Autodesk Inventor part; units mm, degrees
(part 2 of 2)
sketch "Sketch25" plane through (28.3887, -28.3887, -12.2281) normal (0.3845744, -0.3845744, 0.8391693) x (0.7071068, 0.7071068, 0)
  line L0 (-5, 5.9354) -> (-10.5804, 16.196) projected
  line L1 (-5, 0) -> (-5, 5.9354) projected
  line L2 (0, 0) -> (-5, 0) projected
  line L3 (0, 16.196) -> (0, 0) projected
  line L4 (0, 16.196) -> (-10.5804, 16.196) projected
  line L5 (0, 0) -> (5, 0)
  line L6 (0, 0) -> (5, 0) construction
  line L7 (0, 16.196) -> (0, 13.696)
  line L8 (0, 0) -> (0, 1)
  line L9 (0, 1) -> (5, 1)
  line L10 (5, 1) -> (0, 13.696)
  point P0 (0, 40.3412)
  dimension "d119" = 5
  dimension "d120" = 0
  dimension "d121" = 16.196
  dimension "d122" = 2.5
  dimension "d123" = 1
  constraints: 12 end point, 2 horizontal, 2 point on line, 1 collinear, 1 perpendicular
  measures "d119" distance of L2.start L5.end
  measures "d120" distance between parallel lines of L5 L6
  measures "d121" distance of L3.start L2.start
  measures "d122" distance of L3.start L7.end
  measures "d123" distance of L2.start L8.end
extrude "Extrusion25" [suppressed]
sketch "Sketch26" plane through (36.3604, -56.1594, -27.5) normal (0, 0, -1) x (-1, 0, 0)
  line L0 (-6.364, 6.364) -> (38.7544, 51.4823) projected
  line L1 (22.18, 34.9079) -> (23.9685, 35.2898) projected
  line L2 (25.2724, 28.9217) -> (13.7291, 26.457) projected
  line L3 (23.9685, 35.2898) -> (25.3827, 36.704)
  line L4 (13.7291, 26.457) -> (12.3149, 25.0428)
  line L5 (25.2724, 28.9217) -> (26.6866, 27.5075)
  line L6 (24.6794, 37.4073) -> (12.3149, 25.0428)
  line L7 (12.3149, 25.0428) -> (18.2684, 19.0892)
  line L8 (18.2684, 19.0892) -> (30.6329, 31.4538)
  line L9 (30.6329, 31.4538) -> (24.6794, 37.4073)
  line L10 (198.4388, -108.2021) -> (153.3204, -153.3204) projected
  line L11 (24.6794, 37.4073) -> (12.3149, 25.0428)
  line L12 (12.3149, 25.0428) -> (171.9993, -134.6416)
  line L13 (171.9993, -134.6416) -> (184.3638, -122.2771)
  line L14 (184.3638, -122.2771) -> (24.6794, 37.4073)
  point P0 (36.3604, 56.1594)
  point P1 (184.3638, -122.2771)
  point P2 (30.6329, 31.4538)
  point P3 (18.2684, 19.0892)
  dimension "d126" = 2
  dimension "d127" = 2
  dimension "d128" = 2
  constraints: 22 end point, 4 parallel, 2 perpendicular, 2 point on line, 1 collinear
  measures "d126" distance of L1.end L3.end
  measures "d127" distance of L2.end L4.end
  measures "d128" distance of L2.start L5.end
ref_plane "Work Plane11" through (-136.5618, -189.878, -16.0044) normal (-0.3845744, 0.3845744, -0.8391693) x (-0.7071068, -0.7071068, 0)
sketch "Sketch27" plane through (-136.5618, -189.878, -16.0044) normal (-0.3845744, 0.3845744, -0.8391693) x (-0.7071068, -0.7071068, 0)
  line L0 (5, 16.2505) -> (5, 0) projected
  line L1 (5, 16.2505) -> (5, 13.7505)
  line L2 (5, 0) -> (5, 1)
  line L3 (5, 1) -> (10, 1)
  line L4 (10, 1) -> (5, 13.7505)
  point P0 (-230.8278, 40.3412)
  dimension "d131" = 2.5
  dimension "d132" = 1
  dimension "d133" = 5
  dimension "d134" = 90
  constraints: 8 end point, 2 point on line, 1 perpendicular
  measures "d131" distance of L0.start L1.end
  measures "d132" distance of L0.end L2.end
  measures "d133" distance of L2.end L3.end
  measures "d134" angle of L2 L3
ref_plane "Work Plane6" through (23.1226, -30.1936, -16.0044) normal (-0.3845744, 0.3845744, -0.8391693) x (-0.7071068, -0.7071068, 0)
sketch "Sketch28" plane through (23.1226, -30.1936, -16.0044) normal (-0.3845744, 0.3845744, -0.8391693) x (-0.7071068, -0.7071068, 0)
  line L0 (-5, 13.696) -> (-5, 16.2505) projected
  line L1 (-5, 13.696) -> (-10, 1) projected
  line L2 (-5, 16.2505) -> (-4.129, 15.9075)
  line L3 (-5, 16.2505) -> (0, 16.2505) projected
  line L4 (-6.3009, 10.3927) -> (-3.994, 16.2505)
  point P0 (-5, 40.3412)
  point P1 (-5, 13.696)
  constraints: 4 end point, 2 point on line
ref_plane "Work Plane4" through (18.0345, -19.4573, -3.3899) normal (-0.3845744, 0.3845744, -0.8391693) x (-0.5933823, 0.5933823, 0.5438703)
sketch "Sketch29" plane through (18.0345, -19.4573, -3.3899) normal (-0.3845744, 0.3845744, -0.8391693) x (-0.5933823, 0.5933823, 0.5438703)
  line L0 (-0.0545, 1.006) -> (-0.0545, 0.0215) projected
  line L1 (0, 0) -> (-0.0545, 0.0215) projected
  line L2 (0, 1.006) -> (0, 0) projected
  line L3 (-0.0545, 1.006) -> (0, 1.006) projected
  line L4 (-0.0545, -3.994) -> (-17.2505, -3.994) construction
  line L5 (-16.2505, -3.994) -> (-0.0545, -3.994) construction
  line L6 (-0.0545, 1.006) -> (0, 1.006)
  line L7 (0, 1.006) -> (0, -3.994)
  line L8 (0, -3.994) -> (-0.0545, -3.994)
  line L9 (-0.0545, -3.994) -> (-0.0545, 1.006)
  point P0 (24.0907, 1.006)
  constraints: 8 end point, 2 parallel, 1 horizontal, 1 perpendicular
sketch "Sketch31" plane through (-0.9798, 0.9798, -25.5) normal (0.7071068, 0.7071068, 0) x (-0.7071068, 0.7071068, 0)
  line L0 (-27.9421, 22.0804) -> (-28.486, 22.9196) projected
  line L1 (-25.4489, 18.3338) -> (-24.9051, 17.4947) projected
  line L2 (-42.9163, 13.5672) -> (-28.486, 22.9196) projected
  line L3 (-28.486, 22.9196) -> (-28.4402, 22.9493)
  line L4 (-28.4402, 22.9493) -> (-27.8964, 22.1101)
  line L5 (-27.8964, 22.1101) -> (-27.9421, 22.0804)
  line L6 (-27.9421, 22.0804) -> (-28.486, 22.9196)
  point P0 (-1.3856, 25.5)
  point P1 (-27.8964, 22.1101)
  constraints: 8 end point, 2 parallel, 2 perpendicular
ref_plane "Work Plane10" through (23.1226, -30.1936, -16.0044) normal (-0.3845744, 0.3845744, -0.8391693) x (-0.7071068, -0.7071068, 0)
sketch "Sketch32" plane through (23.1226, -30.1936, -16.0044) normal (-0.3845744, 0.3845744, -0.8391693) x (-0.7071068, -0.7071068, 0)
  line L0 (-5, 13.696) -> (-10, 1) projected
  line L1 (-10, 1) -> (-5, 1) projected
  line L2 (-5, 0) -> (-5, 1) projected
  line L3 (-5, 0) -> (0, 0) projected
  line L4 (0, 12.8787) -> (0, 0) projected
  line L5 (-5, 16.2505) -> (1.8338, 16.2505) projected
  line L6 (-5, 13.696) -> (-10, 1) projected
  line L7 (0, 16.2505) -> (0, 0) projected
  line L8 (0, 16.2505) -> (0, 11.2505)
  line L9 (-3.994, 16.2505) -> (-2.494, 16.2505)
  line L10 (-5, 16.2505) -> (0, 16.2505) projected
  line L11 (0, 11.2505) -> (-2.494, 16.2505)
  line L12 (-2.494, 16.2505) -> (-2.494, 11.2505)
  line L13 (-2.494, 16.2505) -> (2.506, 16.2505) construction
  line L14 (-2.494, 11.2505) -> (0, 11.2505)
  line L15 (225.8278, 0) -> (225.8278, 12.8787) projected
  line L16 (225.8278, 0) -> (230.8278, 0) projected
  line L17 (230.8278, 16.2505) -> (230.8278, 0) projected
  line L18 (223.994, 16.2505) -> (230.8278, 16.2505) projected
  line L19 (-5, 13.696) -> (-5, 16.2505) projected
  line L20 (225.8278, 12.8787) -> (223.994, 16.2505) projected
  line L21 (1.8338, 16.2505) -> (0, 12.8787) projected
  point P0 (-5, 40.3412)
  point P1 (-2.494, 16.2505)
  point P2 (0, 11.2505)
  dimension "d144" = 5
  dimension "d145" = 1.5
  dimension "d148" = 5
  dimension "d149" = 90
  constraints: 12 end point, 2 perpendicular, 2 point on line, 1 horizontal
  measures "d144" distance of L7.start L8.end
  measures "d145" distance of L9.start L9.end
  measures "d148" distance of L9.end L12.end
  measures "d149" angle of L12 L13
ref_plane "Work Plane3" through (15.2433, -18.7874, -7.1662) normal (-0.7071068, -0.7071068, 0) x (-0.3845744, 0.3845744, -0.8391693)
sketch "Sketch33" plane through (15.2433, -18.7874, -7.1662) normal (-0.7071068, -0.7071068, 0) x (-0.3845744, 0.3845744, -0.8391693)
  line L0 (-4.5, 0) -> (-4.5, 5) projected
  line L1 (-4.5, 5) -> (0, 5) projected
  line L2 (0, 5) -> (0, 0) projected
  line L3 (-5.5, 0) -> (1, 0) projected
  line L4 (-12.0423, 10.0013) -> (-2.5322, -4.6725) projected
  line L5 (-5.5, 0) -> (-5.5, 17.2505) projected
  line L6 (-5.5, 0) -> (-5.5, -0.0933)
  line L7 (-5.5, 0) -> (-5.4067, 0) construction
  line L8 (1, 0) -> (1, 17.2505) projected
  line L9 (2.9224, -1.1374) -> (-2.5322, -4.6725) projected
  line L10 (1, 0) -> (1, -2.6217)
  line L11 (1, 0) -> (3.6217, 0) construction
  line L12 (2.5, 17.2505) -> (2.5, -1.5)
  line L13 (2.5, -1.5) -> (-7, -1.5)
  line L14 (-7, -1.5) -> (-7, 17.2505)
  point P0 (7.0737, -24.0907)
  point P1 (-4.5883, -1.5)
  point P2 (1, -1.5)
  dimension "d150" = 90
  dimension "d151" = 90
  dimension "d152" = 1.5
  constraints: 14 end point, 2 horizontal, 2 perpendicular, 1 point on line, 2 other
  measures "d150" angle of L6 L7
  measures "d151" angle of L10 L11
  measures "d152" distance between parallel lines of L3 L13
ref_plane "Work Plane8" through (-136.5618, -189.878, -16.0044) normal (-0.3845744, 0.3845744, -0.8391693) x (-0.7071068, -0.7071068, 0)
sketch "Sketch35" plane through (-136.5618, -189.878, -16.0044) normal (-0.3845744, 0.3845744, -0.8391693) x (-0.7071068, -0.7071068, 0)
  line L0 (0, 16.2505) -> (5, 16.2505) projected
  line L1 (5, 16.2505) -> (5, 0) projected
  line L2 (10, 1) -> (5, 13.7505) projected
  line L3 (7.0437, 8.539) -> (4.0196, 16.2505)
  point P0 (-230.8278, 40.3412)
  point P1 (5, 13.7505)
  constraints: 2 end point, 2 point on line
sketch "Sketch36" plane through (-205.4791, -128.0318, -8.9699) normal (-0.7071068, -0.7071068, 0) x (-0.7071068, 0.7071068, 0)
  line L0 (-81.8639, -6.3895) -> (-96.2942, 2.9629) projected
  line L1 (-78.283, -0.9645) -> (-78.8268, -1.8037) projected
  line L2 (-81.8639, -6.3895) -> (-81.32, -5.5503)
  line L3 (-81.32, -5.5503) -> (-81.2742, -5.58)
  line L4 (-81.2742, -5.58) -> (-81.8181, -6.4191)
  line L5 (-81.8181, -6.4191) -> (-81.8639, -6.3895)
  point P0 (-54.7635, -8.9699)
  point P1 (-81.2742, -5.58)
  constraints: 8 end point, 2 parallel, 1 perpendicular
sketch "Sketch37" plane through (-116.96, -209.4798, -27.5) normal (0.7071068, 0.7071068, 0) x (-0.7071068, 0.7071068, 0)
  line L0 (38.9106, 24.1101) -> (34.7148, 21.3907) projected
  line L1 (41.3581, 20.3338) -> (38.9106, 24.1101) projected
  line L2 (37.1622, 17.6145) -> (41.3581, 20.3338) projected
  line L3 (37.1622, 17.6145) -> (34.7148, 21.3907) projected
  point P0 (65.4214, 27.5)
sketch "Sketch38" plane through (-113.5512, 93.7522, -27.5) normal (0, 0, -1) x (-1, 0, 0)
  line L0 (-69.1707, -56.4428) -> (-6.364, 6.364) projected
  line L1 (-21.6597, -8.9317) -> (-23.6391, -19.8047) projected
  line L2 (-30.0242, -18.5868) -> (-29.737, -17.0091) projected
  line L3 (-29.0404, -18.7659) -> (-30.0242, -18.5868) projected
  line L4 (-30.0242, -18.5868) -> (-30.6695, -17.9415)
  line L5 (-30.6695, -17.9415) -> (-31.3766, -18.6487)
  line L6 (-21.6597, -8.9317) -> (-20.9525, -8.2246)
  line L7 (-20.9525, -8.2246) -> (-31.3766, -18.6487)
  line L8 (-31.3766, -18.6487) -> (128.3078, -178.3331)
  line L9 (128.3078, -178.3331) -> (138.7319, -167.909)
  line L10 (138.7319, -167.909) -> (-20.9525, -8.2246)
  point P0 (-113.5512, -93.7522)
  dimension "d174" = 1
  dimension "d175" = 1
  constraints: 14 end point, 3 point on line, 2 parallel, 2 perpendicular, 1 collinear
  measures "d174" distance of L4.end L5.end
  measures "d175" distance of L1.start L6.end
ref_plane "Work Plane7" through (-244.7474, -81.6925, -3.5337) normal (-0.4023607, 0.4023607, 0.8223209) x (0.7071068, 0.7071068, 0)
sketch "Sketch39" plane through (-244.7474, -81.6925, -3.5337) normal (-0.4023607, 0.4023607, 0.8223209) x (0.7071068, 0.7071068, 0)
  line L0 (-5, 0) -> (-5, 16.2505) projected
  line L1 (-5, 16.2505) -> (-5, 15.2505)
  line L2 (-5, 15.2505) -> (-10, 15.2505)
  line L3 (-10, 15.2505) -> (-5, 0)
  line L4 (-5, 15.2505) -> (-5, 14.2505)
  line L5 (-5, 14.2505) -> (-9.6721, 14.2505)
  point P0 (230.8278, -96.8221)
  dimension "d178" = 1
  dimension "d179" = 5
  dimension "d180" = 90
  dimension "d183" = 1
  constraints: 10 end point, 3 point on line, 2 perpendicular
  measures "d178" distance of L0.end L1.end
  measures "d179" distance of L1.end L2.end
  measures "d180" angle of L1 L2
  measures "d183" distance of L1.end L4.end
ref_plane "Work Plane5" through (-81.5274, 81.5274, -3.5337) normal (-0.4023607, 0.4023607, 0.8223209) x (0.7071068, 0.7071068, 0)
sketch "Sketch40" plane through (-81.5274, 81.5274, -3.5337) normal (-0.4023607, 0.4023607, 0.8223209) x (0.7071068, 0.7071068, 0)
  line L0 (0, 16.2505) -> (0, 0) projected
  line L1 (0, 16.2505) -> (-5, 16.2505) projected
  line L2 (0, 16.2505) -> (0, 15.2505)
  line L3 (0, 0) -> (0, 17.2505) projected
  line L4 (0, 15.2505) -> (5, 15.2505)
  line L5 (0, 0) -> (-10.4663, 0) projected
  line L6 (5, 15.2505) -> (0, 0)
  line L7 (0, 15.2505) -> (0, 14.2505)
  line L8 (0, 14.2505) -> (4.6721, 14.2505)
  point P0 (0, -96.8221)
  point P1 (-5, 0)
  point P2 (0, 14.2505)
  dimension "d184" = 1
  dimension "d185" = 5
  dimension "d186" = 90
  dimension "d187" = 1
  constraints: 10 end point, 3 point on line, 2 perpendicular
  measures "d184" distance of L0.start L2.end
  measures "d185" distance of L2.end L4.end
  measures "d186" angle of L4 L2
  measures "d187" distance of L2.end L7.end
sketch "Sketch41" plane through (-107.1872, 100.1162, -9) normal (-0.7071068, -0.7071068, 0) x (-0.7071068, 0.7071068, 0)
  line L0 (-33.8042, -1.7349) -> (-20.4859, 7.481) projected
  line L1 (-31.2884, -5.4663) -> (-17.9253, 3.7806) projected
  line L2 (-34.3732, -0.9125) -> (-33.8042, -1.7349) projected
  line L3 (-35.6067, -1.7661) -> (-34.1841, -3.8219)
  line L4 (-34.1841, -3.8219) -> (-19.6323, 6.2476)
  line L5 (-34.3732, -0.9125) -> (-35.6067, -1.7661)
  line L6 (-35.1718, -2.3945) -> (-32.3309, -6.5)
  line L7 (-20.6314, -6.5) -> (-35.3732, -6.5) projected
  line L8 (-16.5339, 3.5273) -> (-30.7194, -6.2887) projected
  line L9 (-30.07, -5.8393) -> (-31.0248, -6.5)
  line L10 (-35.6067, -1.7661) -> (-31.4951, 1.0791)
  line L11 (-31.4951, 1.0791) -> (-27.7964, -4.266)
  point P0 (-146.5856, -9)
  point P1 (-34.5078, -3.3541)
  dimension "d190" = 1.5
  dimension "d191" = 5
  constraints: 14 end point, 6 point on line, 2 perpendicular, 1 other
  measures "d190" distance between parallel lines of L2 L3
  measures "d191" distance of L3.start L10.end
sketch "Sketch43" plane through (-205.4791, -128.0318, -8.9699) normal (-0.7071068, -0.7071068, 0) x (-0.7071068, 0.7071068, 0)
  line L0 (-95.6027, 3.1105) -> (-16.2332, 125.5744)
  line L1 (-120.1849, 18.5301) -> (-55.3779, 18.5301) projected
  line L2 (-120.1849, -13.9699) -> (-120.1849, 18.5301) projected
  line L3 (91.8221, -13.9699) -> (-120.1849, -13.9699) projected
  line L4 (91.8221, 18.5301) -> (91.8221, -13.9699) projected
  line L5 (2, 18.5301) -> (91.8221, 18.5301) projected
  line L6 (0, 16.5301) -> (2, 18.5301) projected
  line L7 (0, 16.5301) -> (0, 0) projected
  line L8 (0, 0) -> (-5.4, 0) projected
  line L9 (-5.4, 0) -> (-5.4, 16.5301) projected
  line L10 (-7.4, 18.5301) -> (-5.4, 16.5301) projected
  line L11 (-45.9779, 18.5301) -> (-7.4, 18.5301) projected
  line L12 (-47.9779, 16.5301) -> (-45.9779, 18.5301) projected
  line L13 (-47.9779, 16.5301) -> (-47.9779, 0) projected
  line L14 (-47.9779, 0) -> (-53.3779, 0) projected
  line L15 (-53.3779, 0) -> (-53.3779, 16.5301) projected
  line L16 (-55.3779, 18.5301) -> (-53.3779, 16.5301) projected
  line L17 (-100.0531, 9.3651) -> (-100.0531, 4.1651) projected
  line L18 (-100.0531, 4.1651) -> (-110.4531, 4.1651) projected
  line L19 (-110.4531, 4.1651) -> (-110.4531, 9.3651) projected
  arc A0 (-100.0531, 9.3651) -> (-110.4531, 9.3651) centre (-105.2531, 9.3651) ccw projected
  line L20 (77.6221, 4.1651) -> (77.6221, 9.3651) projected
  arc A1 (88.0221, 9.3651) -> (77.6221, 9.3651) centre (82.8221, 9.3651) ccw projected
  line L21 (88.0221, 9.3651) -> (88.0221, 4.1651) projected
  line L22 (88.0221, 4.1651) -> (77.6221, 4.1651) projected
  line L23 (-92.3395, 8.1456) -> (-86.9008, 16.5373)
  line L24 (-86.9008, 16.5373) -> (-72.8443, 7.4271)
  circle A2 centre (-72.8443, 7.4271) radius 1.5
  point P0 (-54.7635, -8.9699)
  dimension "d196" = 10
  dimension "d197" = 3
  constraints: 6 end point, 2 point on line, 1 centre point, 1 coincident, 1 perpendicular, 3 other
  measures "d196" distance of L23.start L23.end
  measures "d197" diameter of A2
extrude "Extrusion41" cut sketch "Sketch43" against normal through all contours A2
sketch "Sketch44" plane through (-205.4791, -128.0318, -8.9699) normal (-0.7071068, -0.7071068, 0) x (-0.7071068, 0.7071068, 0)
  line L0 (73.3581, 2.8319) -> (49.1605, 37.8849)
  line L1 (57.4489, -0.8824) -> (71.5895, 8.9025) projected
  line L2 (69.9504, 7.7683) -> (64.2694, 15.9979)
  line L3 (64.2694, 15.9979) -> (51.7041, 7.3238)
  circle A0 centre (51.7041, 7.3238) radius 1.5
  line L4 (51.7041, 7.3238) -> (50.8811, 6.7557)
  circle A1 centre (50.8811, 6.7557) radius 1.5
  line L5 (50.8811, 6.7557) -> (50.4697, 6.4717)
  circle A2 centre (50.4697, 6.4717) radius 1.5
  line L6 (51.7041, 7.3238) -> (47.8105, 7.3238)
  line L7 (50.4697, 6.4717) -> (50.4697, 7.3238)
  line L8 (50.4697, 6.4717) -> (64.2694, 15.9979)
  circle A3 centre (49.8814, 7.3238) radius 1.5
  point P0 (-54.7635, -8.9699)
  dimension "d202" = 3
  dimension "d200" = 10
  dimension "d201" = 90
  dimension "d205" = 1
  dimension "d206" = 3
  dimension "d207" = 0.5
  dimension "d208" = 3
  dimension "d210" = 16.7685
  dimension "d211" = 3
  constraints: 16 end point, 5 point on line, 3 centre point, 3 coincident, 1 collinear, 1 horizontal, 1 perpendicular, 6 other
  measures "d200" distance of L2.start L2.end
  measures "d201" angle of L3 L2
  measures "d205" distance of L4.start L4.end
  measures "d206" diameter of A1
  measures "d207" distance of L5.start L5.end
  measures "d208" diameter of A2
  measures "d210" distance of L2.end L5.end
  measures "d211" diameter of A3
extrude "Extrusion42" cut sketch "Sketch44" against normal through all contours A3 A1 A0 | A0 A1 A2 L6 A3 | A3 A2 A0 A1 | A0 A2 A1 | L6 A2 A3 | A3 A0 L5 L4 | L4 L5 L7 L6 A3 | A3 L6 A0 A2 | A0 L6 A1 A2 | A1 L6 A2 | L6 A1 A3 A2 | A3 A1 L6 A0 | L7 A0 L6 picked at (50.8658, 8.0245) picked at (50.2576, 8.0086) picked at (48.8997, 7.2299)
sketch "Sketch45" plane through (-0.9798, 0.9798, -25.5) normal (0.7071068, 0.7071068, 0) x (-0.7071068, 0.7071068, 0)
  circle A0 centre (103.2593, 9.2063) radius 1.5
  line L0 (91.1129, 7.8859) -> (91.5834, 10.0898)
  line L1 (89.5634, -0.0795) -> (91.1184, 7.8847)
  line L2 (89.2936, 10.0898) -> (84.3438, 5.14)
  line L3 (89.5634, -0.0795) -> (91.7684, -2.2846)
  line L4 (84.3438, 5.14) -> (89.5634, -0.0795)
  line L5 (89.2936, 10.0898) -> (91.5834, 10.0898)
  line L6 (91.5834, 10.0898) -> (94.2433, 10.0898)
  circle A1 centre (103.2593, 9.2063) radius 11.7092
  circle A2 centre (103.2593, 9.2063) radius 10.7092
  circle A3 centre (103.2593, 9.2063) radius 19.3476
  circle A4 centre (103.2593, 9.2063) radius 20.3476
  line L7 (89.2098, -0.4331) -> (83.6367, 5.14)
  line L8 (83.6367, 5.14) -> (89.0865, 10.5898)
  line L9 (89.0865, 10.5898) -> (91.5834, 10.5898)
  line L10 (98.3095, 14.156) -> (94.2433, 10.0898)
  line L11 (89.0865, 10.5898) -> (94.7433, 10.5898)
  line L12 (89.0865, 10.5898) -> (83.3769, 4.8802)
  line L13 (145.2, -2) -> (55.3779, -2) projected
  line L14 (103.2593, 9.2063) -> (103.2593, -2.503)
  line L15 (103.2593, -1.503) -> (106.6542, -1.503)
  line L16 (145.2, -2) -> (56.3779, -2) projected
  line L17 (106.6542, -2) -> (106.6542, -1.503)
  point P0 (-1.3856, 25.5)
  point P1 (92.6398, 10.5898)
  point P2 (83.6367, 5.14)
  point P3 (86.2756, -2)
  point P4 (99.8643, -2)
  dimension "d213" = 1
  dimension "d212" = 1
  dimension "d214" = 0.5
  constraints: 32 end point, 5 point on line, 3 horizontal, 3 point on circle, 2 centre point, 2 coincident, 2 perpendicular, 1 parallel, 28 other
  measures "d214" distance between parallel lines of L2 L8
extrude "Extrusion43" cut sketch "Sketch45" against normal through all contours L5 A1 L13 L3 L4 L2 | L2 A3 L8 L9 L11 A1 L5 | A3 L7 L8 | L4 L3 L13 A3 | A1 L11 A2 L6 | L6 A2 L14 L13 A1 | A3 L13 A4 L12 L7 | L13 L14 A1 | L15 L17 L13 L14 | L14 L13 A1
sketch "Sketch46" plane through (-0.9798, 0.9798, -25.5) normal (0.7071068, 0.7071068, 0) x (-0.7071068, 0.7071068, 0)
  circle A0 centre (-19.4664, 9.103) radius 1.5
  line L0 (-5.7825, -0.2006) -> (-7.3272, 7.7657)
  line L1 (-7.3217, 7.7668) -> (-7.7894, 9.9713)
  line L2 (-5.4995, 9.9684) -> (-7.7894, 9.9713)
  line L3 (-5.4995, 9.9684) -> (-0.5562, 5.0122)
  line L4 (-0.5562, 5.0122) -> (-5.7825, -0.2006)
  line L5 (-8.309, 7.5753) -> (-6.4066, -2.2354)
  line L6 (-6.4066, -2.2354) -> (0.858, 5.0104)
  line L7 (0.858, 5.0104) -> (-5.084, 10.9678)
  line L8 (-5.084, 10.9678) -> (-9.0242, 10.9729)
  line L9 (-9.0242, 10.9729) -> (-8.2999, 7.5593)
  circle A1 centre (-19.4664, 9.103) radius 10.6083
  line L10 (-2, -2) -> (-66.807, -2) projected
  line L11 (-19.4664, 9.103) -> (-19.4664, -2)
  line L12 (-19.4664, -1.5054) -> (-22.8614, -1.5054)
  line L13 (-22.8614, -1.5054) -> (-22.8614, -2)
  line L14 (0, 0) -> (-2, -2) projected
  line L15 (0, 0) -> (0, 16.5301) projected
  point P0 (-1.3856, 25.5)
  point P1 (0, 5.8706)
  dimension "d217" = 1
  dimension "d218" = 3.395
  constraints: 26 end point, 3 point on line, 2 centre point, 2 perpendicular, 2 point on circle, 1 coincident, 1 horizontal, 1 tangent, 17 other
  measures "d217" distance between parallel lines of L0 L5
  measures "d218" distance of L12.start L12.end
extrude "Extrusion44" cut sketch "Sketch46" against normal through all contours L10 L11 A1 L8 L7 L15 L6 | L6 L15 L14 L10 | L10 L13 L12 L11
sketch "Sketch47" plane through (-266.8716, -59.5682, -27.5) normal (0.7071068, 0.7071068, 0) x (-0.7071068, 0.7071068, 0)
  line L0 (-14.2, 9.1651) -> (-14.2, 14.3651) projected
  line L1 (-14.2, 14.3651) -> (-3.8, 14.3651) projected
  line L2 (-3.8, 14.3651) -> (-3.8, 9.1651) projected
  arc A0 (-14.2, 9.1651) -> (-3.8, 9.1651) centre (-9, 9.1651) ccw projected
  arc A1 (-61.8231, 6.8802) -> (-58.9244, 0) centre (-41.9407, 11.2063) ccw projected
  line L3 (-61.8231, 6.8802) -> (-56.1135, 12.5898) projected
  line L4 (-56.1135, 12.5898) -> (-52.5602, 12.5898) projected
  arc A2 (-52.5602, 12.5898) -> (-41.9407, 0.497) centre (-41.9407, 11.2063) ccw projected
  line L5 (-41.9407, 0.497) -> (-38.5458, 0.497) projected
  line L6 (-38.5458, 0.497) -> (-38.5458, 0) projected
  line L7 (0, 0) -> (-38.5458, 0) projected
  line L8 (0, 18.5) -> (0, 0) projected
  line L9 (-88.8221, 18.5) -> (0, 18.5) projected
  line L10 (-88.8221, 18.5) -> (-88.8221, 0) projected
  line L11 (-58.9244, 0) -> (-88.8221, 0) projected
  circle A3 centre (-41.9407, 11.2063) radius 1.5 projected
  arc A4 (-63.9864, 7.5454) -> (-62.3039, 2) centre (-41.9407, 11.2063) ccw
  line L12 (-63.9864, 7.5454) -> (-56.942, 14.5898)
  line L13 (-56.942, 14.5898) -> (-49.9658, 14.5898)
  arc A5 (-49.9658, 14.5898) -> (-41.9407, 2.497) centre (-41.9407, 11.2063) ccw
  line L14 (-41.9407, 2.497) -> (-36.5458, 2.497)
  line L15 (-36.5458, 2.497) -> (-36.5458, 2)
  line L16 (-2, 2) -> (-2, 16.5)
  line L17 (-2, 16.5) -> (-86.8221, 16.5)
  line L18 (-86.8221, 16.5) -> (-86.8221, 2)
  line L19 (-86.8221, 2) -> (-66.7033, 2)
  line L20 (-36.5458, 2.497) -> (-36.5458, 0)
  line L21 (-36.5458, 2) -> (-36.4697, 2)
  line L22 (-23.7949, 2) -> (-2, 2)
  arc A6 (-63.9864, 7.5454) -> (-61.2755, 0) centre (-41.9407, 11.2063) ccw
  arc A7 (-22.6059, 0) -> (-63.6523, 16.5) centre (-41.9407, 11.2063) ccw
  line L23 (-168.0614, 0) -> (-168.0614, 0.4946) projected
  line L24 (-168.0614, 0.4946) -> (-164.6664, 0.4946) projected
  arc A8 (-164.6664, 0.4946) -> (-154.2242, 12.9729) centre (-164.6664, 11.103) ccw projected
  line L25 (-154.2242, 12.9729) -> (-150.284, 12.9678) projected
  line L26 (-150.284, 12.9678) -> (-148.2, 10.8784) projected
  line L27 (-148.2, 10.8784) -> (-148.2, 18.5) projected
  line L28 (-212.007, 18.5) -> (-148.2, 18.5) projected
  line L29 (-212.007, 0) -> (-212.007, 18.5) projected
  line L30 (-168.0614, 0) -> (-212.007, 0) projected
  line L31 (-191.8753, 14.3651) -> (-191.8753, 9.1651) projected
  arc A9 (-202.2753, 9.1651) -> (-191.8753, 9.1651) centre (-197.0753, 9.1651) ccw projected
  line L32 (-202.2753, 9.1651) -> (-202.2753, 14.3651) projected
  line L33 (-202.2753, 14.3651) -> (-191.8753, 14.3651) projected
  circle A10 centre (-164.6664, 11.103) radius 1.5 projected
  arc A11 (-164.6664, 2.4946) -> (-156.9788, 14.9765) centre (-164.6664, 11.103) ccw
  line L34 (-164.6664, 2.4946) -> (-170.0614, 2.4946)
  line L35 (-170.0614, 2.4946) -> (-170.0614, 2)
  line L36 (-170.0614, 2) -> (-210.007, 2)
  line L37 (-210.007, 2) -> (-210.007, 16.5)
  line L38 (-210.007, 16.5) -> (-150.2, 16.5)
  line L39 (-150.2, 16.5) -> (-150.2, 14.9677)
  line L40 (-150.2, 14.9677) -> (-156.9788, 14.9765)
  line L41 (-170.0614, 2.4946) -> (-170.0614, 0)
  line L42 (-150.2, 14.9677) -> (-144.1267, 8.8787)
  line L43 (-150.284, 12.9678) -> (-148.2, 10.8784) projected
  point P0 (-146.5856, 27.5)
  point P1 (-36.5458, 2)
  point P2 (-62.3039, 2)
  point P3 (-148.2, 12.9625)
  point P4 (-170.0614, 2)
  dimension "d221" = 2
  dimension "d224" = 2
  constraints: 40 end point, 12 point on circle, 6 point on line, 5 centre point, 1 coincident, 1 parallel, 1 perpendicular, 1 vertical, 14 other
  measures "d221" radial gap between concentric circles of A1 A4
  measures "d224" radial gap between concentric circles of A8 A11
extrude "Extrusion45" add sketch "Sketch47" along normal up to surface (3 mm away) contours A1 L11 A6 A4 L12 L13 A5 L14 L15 L20 L7 L6 L5 A2 L4 L3 | L30 L41 L35 L34 A11 L40 L42 L27 L26 L25 A8 L24 L23
sketch "Sketch48" plane through (-107.1872, 100.1162, -9) normal (-0.7071068, -0.7071068, 0) x (-0.7071068, 0.7071068, 0)
  line L0 (-145.2, 10.6294) -> (-150.284, 5.5322) projected
  line L1 (-145.2, 10.6294) -> (-145.2, -0.0301) projected
  line L2 (-145.2, -0.0301) -> (-139.8, -0.0301) projected
  line L3 (-139.8, -0.0301) -> (-139.8, 16.5) projected
  line L4 (-139.8, 16.5) -> (-137.8, 18.5) projected
  line L5 (-137.8, 18.5) -> (-136.8, 18.5) projected
  line L6 (-136.8, 18.5) -> (-136.8, -3) projected
  line L7 (-148.2, -3) -> (-136.8, -3) projected
  line L8 (-148.2, -3) -> (-148.2, 5.5375) projected
  line L9 (-150.2, 3.5323) -> (-148.2, 5.5375) projected
  line L10 (-156.9788, 3.5235) -> (-150.2, 3.5323) projected
  arc A0 (-156.9788, 3.5235) -> (-164.6664, 16.0054) centre (-164.6664, 7.397) ccw projected
  line L11 (-170.0614, 16.0054) -> (-164.6664, 16.0054) projected
  line L12 (-170.0614, 18.5) -> (-170.0614, 16.0054) projected
  line L13 (-168.0614, 18.5) -> (-170.0614, 18.5) projected
  line L14 (-168.0614, 18.0054) -> (-168.0614, 18.5) projected
  line L15 (-164.6664, 18.0054) -> (-168.0614, 18.0054) projected
  arc A1 (-154.2242, 5.5271) -> (-164.6664, 18.0054) centre (-164.6664, 7.397) ccw projected
  line L16 (-150.284, 5.5322) -> (-154.2242, 5.5271) projected
  line L17 (-38.5458, 18.5) -> (-38.5458, 18.003) projected
  line L18 (-36.5458, 18.5) -> (-38.5458, 18.5) projected
  line L19 (-36.5458, 16.003) -> (-36.5458, 18.5) projected
  line L20 (-41.9407, 16.003) -> (-36.5458, 16.003) projected
  arc A2 (-41.9407, 16.003) -> (-49.9658, 3.9102) centre (-41.9407, 7.2937) ccw projected
  line L21 (-56.942, 3.9102) -> (-49.9658, 3.9102) projected
  line L22 (-63.9864, 10.9546) -> (-56.942, 3.9102) projected
  arc A3 (-61.2755, 18.5) -> (-63.9864, 10.9546) centre (-41.9407, 7.2937) ccw projected
  line L23 (-58.9244, 18.5) -> (-61.2755, 18.5) projected
  arc A4 (-58.9244, 18.5) -> (-61.8231, 11.6198) centre (-41.9407, 7.2937) ccw projected
  line L24 (-56.1135, 5.9102) -> (-61.8231, 11.6198) projected
  line L25 (-52.5602, 5.9102) -> (-56.1135, 5.9102) projected
  arc A5 (-41.9407, 18.003) -> (-52.5602, 5.9102) centre (-41.9407, 7.2937) ccw projected
  line L26 (-38.5458, 18.003) -> (-41.9407, 18.003) projected
  point P0 (-146.5856, -9)
extrude "Extrusion46" add sketch "Sketch48" along normal blind 2
chamfer "Chamfer4" distance 2 angle 45 16 edges at (-232.0838, -94.356, -21.1095) (-239.1225, -87.3174, -25.003) (-229.074, -97.3659, -12.9102) (-224.117, -102.3229, -16.4324) (-64.4326, 57.3615, -16.4324) (-69.3896, 62.3185, -12.9102) (-72.3994, 65.3284, -21.1095) (-79.4381, 72.367, -25.003) (4.0666, -11.1377, -20.9114) (11.1569, -18.228, -25.0054) (1.4169, -8.4879, -12.5279) (-1.6869, -5.3842, -13.5349) (-155.6178, -170.8221, -20.9114) (-148.5275, -177.9124, -25.0054) (-158.2675, -168.1723, -12.5279) (-161.3713, -165.0686, -13.5349)
sketch "Sketch49" plane through (-177.7565, 49.3459, -21.4172) normal (-0.7071068, 0.7071068, 0) x (-0.7071068, -0.7071068, 0)
  line L0 (-76.8, 26.4172) -> (131.0278, 26.4172) projected
  line L1 (-76.8, 24.4172) -> (131.0278, 24.4172)
  line L2 (131.0278, 26.4172) -> (129.0278, 24.4172)
  line L3 (131.0278, 26.4172) -> (133.8563, 26.4172) construction
  line L4 (129.0278, 24.4172) -> (124.0278, 24.4172)
  line L5 (129.0278, 24.4172) -> (127.0278, 26.4172)
  line L6 (129.0278, 24.4172) -> (131.8563, 24.4172) construction
  line L7 (127.0278, 26.4172) -> (122.0278, 26.4172)
  line L8 (122.0278, 26.4172) -> (120.0278, 24.4172)
  line L9 (120.0278, 24.4172) -> (118.0278, 26.4172)
  line L10 (118.0278, 26.4172) -> (113.0278, 26.4172)
  line L11 (113.0278, 26.4172) -> (111.0278, 24.4172)
  line L12 (111.0278, 24.4172) -> (109.0278, 26.4172)
  line L13 (111.0278, 24.4172) -> (113.8563, 24.4172) construction
  line L14 (109.0278, 26.4172) -> (104.0278, 26.4172)
  line L15 (104.0278, 26.4172) -> (102.0278, 24.4172)
  line L16 (102.0278, 24.4172) -> (100.0278, 26.4172)
  line L17 (100.0278, 26.4172) -> (95.0278, 26.4172)
  line L18 (95.0278, 26.4172) -> (93.0278, 24.4172)
  line L19 (93.0278, 24.4172) -> (91.0278, 26.4172)
  line L20 (101.7528, 26.4172) -> (-50.3403, 26.4172) projected
  line L21 (91.0278, 26.4172) -> (86.0278, 26.4172)
  line L22 (86.0278, 26.4172) -> (84.0278, 24.4172)
  line L23 (84.0278, 24.4172) -> (82.0278, 26.4172)
  line L24 (71.7094, 26.4172) -> (82.5838, 26.4172) projected
  line L25 (82.0278, 26.4172) -> (77.0278, 26.4172)
  line L26 (77.0278, 26.4172) -> (75.0278, 24.4172)
  line L27 (75.0278, 24.4172) -> (73.0278, 26.4172)
  line L28 (73.0278, 26.4172) -> (68.0278, 26.4172)
  line L29 (68.0278, 26.4172) -> (66.0278, 24.4172)
  line L30 (66.0278, 24.4172) -> (64.0278, 26.4172)
  line L31 (64.0278, 26.4172) -> (59.0278, 26.4172)
  line L32 (59.0278, 26.4172) -> (57.0278, 24.4172)
  line L33 (57.0278, 24.4172) -> (55.0278, 26.4172)
  line L34 (55.0278, 26.4172) -> (50.0278, 26.4172)
  line L35 (50.0278, 26.4172) -> (48.0278, 24.4172)
  line L36 (48.0278, 24.4172) -> (46.0278, 26.4172)
  line L37 (46.0278, 26.4172) -> (41.0278, 26.4172)
  line L38 (41.0278, 26.4172) -> (39.0278, 24.4172)
  line L39 (39.0278, 24.4172) -> (37.0278, 26.4172)
  line L40 (37.0278, 26.4172) -> (32.0278, 26.4172)
  line L41 (32.0278, 26.4172) -> (30.0278, 24.4172)
  line L42 (-76.8, 26.4172) -> (-74.8, 24.4172)
  line L43 (-76.8, 26.4172) -> (-73.9716, 26.4172) construction
  line L44 (-74.8, 24.4172) -> (-72.8, 26.4172)
  line L45 (-72.8, 26.4172) -> (-67.8, 26.4172)
  line L46 (-67.8, 26.4172) -> (-65.8, 24.4172)
  line L47 (-65.8, 24.4172) -> (-63.8, 26.4172)
  line L48 (-63.8, 26.4172) -> (-58.8, 26.4172)
  line L49 (-58.8, 26.4172) -> (-56.8, 24.4172)
  line L50 (-56.8, 24.4172) -> (-54.8, 26.4172)
  line L51 (-54.8, 26.4172) -> (-49.8, 26.4172)
  line L52 (-49.8, 26.4172) -> (-47.8, 24.4172)
  line L53 (-47.8, 24.4172) -> (-45.8, 26.4172)
  line L54 (-45.8, 26.4172) -> (-40.8, 26.4172)
  line L55 (-40.8, 26.4172) -> (-38.8, 24.4172)
  line L56 (-38.8, 24.4172) -> (-36.8, 26.4172)
  line L57 (-36.8, 26.4172) -> (-31.8, 26.4172)
  line L58 (-31.8, 26.4172) -> (-29.8, 24.4172)
  line L59 (-29.8, 24.4172) -> (-27.8, 26.4172)
  line L60 (-27.8, 26.4172) -> (-22.8, 26.4172)
  line L61 (-22.8, 26.4172) -> (-20.8, 24.4172)
  line L62 (-20.8, 24.4172) -> (-18.8, 26.4172)
  line L63 (-18.8, 26.4172) -> (-13.8, 26.4172)
  line L64 (-13.8, 26.4172) -> (-11.8, 24.4172)
  line L65 (-11.8, 24.4172) -> (-9.8, 26.4172)
  line L66 (-9.8, 26.4172) -> (-4.8, 26.4172)
  line L67 (-4.8, 26.4172) -> (-2.8, 24.4172)
  line L68 (-2.8, 24.4172) -> (-0.8, 26.4172)
  line L69 (-0.8, 26.4172) -> (4.2, 26.4172)
  line L70 (4.2, 26.4172) -> (6.2, 24.4172)
  line L71 (6.2, 24.4172) -> (8.2, 26.4172)
  line L72 (8.2, 26.4172) -> (13.2, 26.4172)
  line L73 (13.2, 26.4172) -> (15.2, 24.4172)
  line L74 (15.2, 24.4172) -> (17.2, 26.4172)
  line L75 (17.2, 26.4172) -> (22.2, 26.4172)
  line L76 (22.2, 26.4172) -> (24.2, 24.4172)
  point P0 (-90.8, 21.4172)
  point P1 (-45.8, 26.4172)
  point P2 (-49.8, 26.4172)
  point P3 (-36.8, 26.4172)
  point P4 (-40.8, 26.4172)
  point P5 (-27.8, 26.4172)
  point P6 (-31.8, 26.4172)
  point P7 (-18.8, 26.4172)
  point P8 (-22.8, 26.4172)
  point P9 (-9.8, 26.4172)
  point P10 (-13.8, 26.4172)
  point P11 (-0.8, 26.4172)
  point P12 (-4.8, 26.4172)
  point P13 (8.2, 26.4172)
  point P14 (4.2, 26.4172)
  point P15 (17.2, 26.4172)
  point P16 (13.2, 26.4172)
  point P17 (77.0278, 26.4172)
  point P18 (82.0278, 26.4172)
  point P19 (91.0278, 26.4172)
  dimension "d230" = 2
  dimension "d231" = 135
  dimension "d232" = 5
  dimension "d233" = 135
  dimension "d234" = 5
  dimension "d235" = 135
  dimension "d236" = 90
  dimension "d237" = 5
  dimension "d238" = 135
  dimension "d239" = 5
  dimension "d240" = 135
  dimension "d241" = 90
  dimension "d242" = 5
  dimension "d243" = 135
  dimension "d244" = 90
  dimension "d245" = 5
  dimension "d246" = 135
  dimension "d247" = 90
  dimension "d248" = 5
  dimension "d249" = 135
  dimension "d250" = 90
  dimension "d251" = 5
  dimension "d252" = 135
  dimension "d253" = 90
  dimension "d254" = 5
  dimension "d255" = 135
  dimension "d256" = 90
  dimension "d257" = 5
  dimension "d258" = 135
  dimension "d259" = 90
  dimension "d260" = 5
  dimension "d261" = 135
  dimension "d262" = 90
  dimension "d263" = 5
  dimension "d264" = 135
  dimension "d265" = 45
  dimension "d266" = 90
  dimension "d267" = 5
  dimension "d268" = 135
  dimension "d269" = 90
  dimension "d270" = 5
  dimension "d271" = 135
  dimension "d272" = 90
  dimension "d273" = 5
  dimension "d274" = 135
  dimension "d275" = 90
  dimension "d276" = 5
  dimension "d277" = 135
  dimension "d278" = 90
  dimension "d279" = 5
  dimension "d280" = 135
  dimension "d281" = 90
  dimension "d282" = 5
  dimension "d283" = 135
  dimension "d284" = 90
  dimension "d285" = 5
  dimension "d286" = 135
  dimension "d287" = 90
  dimension "d288" = 5
  dimension "d289" = 135
  dimension "d290" = 90
  dimension "d291" = 5
  dimension "d292" = 135
  dimension "d293" = 90
  dimension "d294" = 5
  constraints: 146 end point, 4 equal length, 4 horizontal, 2 point on line, 1 perpendicular, 72 other
  measures "d231" angle of L2 L3
  measures "d232" distance of L2.end L4.end
  measures "d233" angle of L6 L5
  measures "d234" distance of L5.end L7.end
  measures "d235" angle of L8 L7
  measures "d236" angle of L8 L9
  measures "d237" distance of L9.end L10.end
  measures "d238" angle of L13 L12
  measures "d239" distance of L12.end L14.end
  measures "d240" angle of L15 L14
  measures "d241" angle of L15 L16
  measures "d242" distance of L16.end L17.end
  measures "d243" angle of L18 L17
  measures "d244" angle of L18 L19
  measures "d245" distance of L19.end L21.end
  measures "d246" angle of L22 L21
  measures "d247" angle of L22 L23
  measures "d248" distance of L23.end L25.end
  measures "d249" angle of L26 L25
  measures "d250" angle of L26 L27
  measures "d251" distance of L27.end L28.end
  measures "d252" angle of L29 L28
  measures "d253" angle of L29 L30
  measures "d254" distance of L30.end L31.end
  measures "d255" angle of L32 L31
  measures "d256" angle of L32 L33
  measures "d257" distance of L33.end L34.end
  measures "d258" angle of L35 L34
  measures "d259" angle of L35 L36
  measures "d260" distance of L36.end L37.end
  measures "d261" angle of L38 L37
  measures "d262" angle of L38 L39
  measures "d263" distance of L39.end L40.end
  measures "d264" angle of L41 L40
  measures "d265" angle of L42 L43
  measures "d266" angle of L44 L42
  measures "d267" distance of L44.end L45.end
  measures "d268" angle of L45 L46
  measures "d269" angle of L47 L46
  measures "d270" distance of L47.end L48.end
  measures "d271" angle of L48 L49
  measures "d272" angle of L50 L49
  measures "d273" distance of L50.end L51.end
  measures "d274" angle of L51 L52
  measures "d275" angle of L53 L52
  measures "d276" distance of L53.end L54.end
  measures "d277" angle of L54 L55
  measures "d278" angle of L56 L55
  measures "d279" distance of L56.end L57.end
  measures "d280" angle of L57 L58
  measures "d281" angle of L59 L58
  measures "d282" distance of L59.end L60.end
  measures "d283" angle of L60 L61
  measures "d284" angle of L62 L61
  measures "d285" distance of L62.end L63.end
  measures "d286" angle of L63 L64
  measures "d287" angle of L65 L64
  measures "d288" distance of L65.end L66.end
  measures "d289" angle of L66 L67
  measures "d290" angle of L68 L67
  measures "d291" distance of L68.end L69.end
  measures "d292" angle of L69 L70
  measures "d293" angle of L71 L70
  measures "d294" distance of L71.end L72.end
extrude "Extrusion47" cut sketch "Sketch49" against normal through all contours L0 L44 L42 | L0 L47 L46 | L49 L0 L50 | L52 L0 L53 | L55 L0 L56 | L58 L0 L59 | L61 L0 L62 | L64 L0 L65 | L67 L0 L68 | L70 L0 L71 | L73 L0 L74 | L76 L0 L41 L1 | L39 L0 L38 | L36 L0 L35 | L33 L0 L32 | L30 L0 L29 | L27 L0 L26 | L23 L0 L22 | L19 L0 L18 | L16 L0 L15 | L12 L0 L11 | L9 L0 L8 | L5 L0 L2
sketch "Sketch50" plane through (0, 0, 5) normal (0, 0, 1) x (1, 0, 0)
  circle A0 centre (-155.6221, -117.443) radius 3.25 projected
  circle A1 centre (-155.6221, -117.443) radius 1.5 projected
  circle A2 centre (-155.6221, -117.443) radius 6.25
  circle A3 centre (-101.5774, -63.4504) radius 3.25 projected
  circle A4 centre (-101.5774, -63.4504) radius 1.5 projected
  circle A5 centre (-48.5978, -10.4708) radius 3.25 projected
  circle A6 centre (-48.5978, -10.4708) radius 1.5 projected
  circle A7 centre (-48.5978, -10.4708) radius 6.25
  circle A8 centre (-101.5774, -63.4504) radius 6.25
  point P0 (0, 0)
  dimension "d301" = 3
  dimension "d302" = 3
  dimension "d303" = 3
  constraints: 3 centre point
  measures "d301" radial gap between concentric circles of A0 A2
  measures "d302" radial gap between concentric circles of A5 A7
  measures "d303" radial gap between concentric circles of A3 A8
extrude "Extrusion48" add sketch "Sketch50" against normal blind 2 contours A2 | A7 | A8
sketch "Sketch51" plane through (0, 0, 5) normal (0, 0, 1) x (1, 0, 0)
  circle A0 centre (39.8249, -56.1594) radius 1.5 projected
  circle A1 centre (-113.5512, 97.2167) radius 1.5 projected
  circle A2 centre (-263.9721, -53.2043) radius 1.5 projected
  circle A3 centre (-110.5961, -206.5803) radius 1.5 projected
  arc A4 (-120.4956, -213.0154) -> (-100.6966, -213.0154) centre (-110.5961, -203.1159) ccw projected
  line L0 (-107.7676, -193.2164) -> (-110.5961, -196.0448) projected
  circle A5 centre (-110.5961, -206.5803) radius 10.5355
  circle A6 centre (39.8249, -56.1594) radius 10.5355
  circle A7 centre (-113.5512, 97.2167) radius 10.5355
  circle A8 centre (-263.9721, -53.2043) radius 10.5389
  point P0 (0, 0)
  point P1 (-113.5512, 86.6811)
  constraints: 4 coincident, 2 centre point, 2 vertical alignment, 4 other
extrude "Extrusion49" add sketch "Sketch51" against normal blind 2
body "Solid1"
